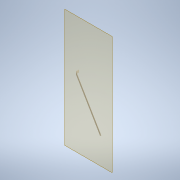
# Autodesk Inventor part: cover_inside_support_1
Saved by Autodesk Inventor 2021 (Build 250183000, 183)
## iProperties
Created: 2021-06-25
Part Number: cover_inside_support_1
Material: Generic
Document SubType Name: Modeling
Density: 1 g/cm^3
Appearance: Default
Autodesk Inventor part; units mm, degrees
ref_plane "YZ Plane" through (0, 0, 0) normal (1, 0, 0) x (0, 1, 0)
ref_plane "XZ Plane" through (0, 0, 0) normal (0, 1, 0) x (-1, 0, 0)
ref_plane "XY Plane" through (0, 0, 0) normal (0, 0, 1) x (1, 0, 0)
ref_plane "Work Plane1" through (0, 0, 0) normal (0, 0, 1) x (1, 0, 0)
sketch "Sketch1" plane through (0, 0, 0) normal (0, 0, 1) x (1, 0, 0)
  line L0 (180, 1409.2846) -> (716.3958, 495.0201)
  line L1 (180, 1350) -> (690.5204, 479.8391)
  line L2 (716.3958, 495.0201) -> (690.5204, 479.8391)
  line L3 (180, 1409.2846) -> (180, 1350)
  point P0 (0, 0)
  dimension "d0" = 30
  dimension "d2" = 180
  dimension "d3" = 1350
  dimension "d4" = 149.6
  dimension "d5" = 1060
  constraints: 8 end point, 2 perpendicular, 1 vertical
  measures "d0" distance of L0.end L1.end
  measures "d2" distance from line of point (0, 0) L3
  measures "d3" vertical distance of point (0, 0) L1.start
  measures "d4" angle of L1 L3
  measures "d5" distance of L0.start L0.end
extrude "Extrusion1" add sketch "Sketch1" against normal blind 6
sketch "Sketch2" plane through (0, 0, 0) normal (0, 0, 1) x (1, 0, 0)
  line L0 (843.3143, 1707.8077) -> (86.6419, 1707.8077)
  line L1 (86.6419, 1707.8077) -> (86.6419, 311.9107)
  line L2 (86.6419, 311.9107) -> (843.3143, 311.9107)
  line L3 (843.3143, 311.9107) -> (843.3143, 1707.8077)
  point P0 (0, 0)
  constraints: 8 end point, 2 parallel, 1 horizontal, 1 perpendicular
extrude "Extrusion2" cut sketch "Sketch2" against normal blind 3
sketch "Sketch3" plane through (0, 0, -6) normal (0, 0, -1) x (-1, 0, 0)
  line L0 (-690.5204, 479.8391) -> (-180, 1350) projected
  line L1 (-183.1729, 1344.5919) -> (-186.1729, 1344.5919)
  line L2 (-186.1729, 1344.5919) -> (-186.1729, 1403.4543)
  line L3 (-186.1729, 1403.4543) -> (-183.1729, 1403.4543)
  line L4 (-183.1729, 1403.4543) -> (-183.1729, 1344.5919)
  point P0 (0, 0)
  dimension "d10" = 3
  constraints: 8 end point, 2 parallel, 1 horizontal, 1 perpendicular, 1 point on line
  measures "d10" distance between parallel lines of L2 L4
extrude "Extrusion3" add sketch "Sketch3" along normal blind 60
fillet "Fillet1" radius 6 2 edges at (716.3958, 495.0201, -4.5) (690.5204, 479.8391, -4.5)
sketch "Sketch4" plane through (0, 0, -6) normal (0, 0, -1) x (-1, 0, 0)
  line L0 (-183.1729, 1403.4543) -> (-183.1729, 1344.5919) projected
  line L1 (-183.1729, 1403.4543) -> (-183.1729, 1344.5919)
  line L2 (-183.1729, 1403.4543) -> (-186.6492, 1397.5292)
  line L3 (-180, 1409.2846) -> (-183.4206, 1403.4543) projected
  line L4 (-186.6492, 1397.5292) -> (-186.6492, 1414.0356)
  line L5 (-186.6492, 1414.0356) -> (-167.7898, 1414.0356)
  line L6 (-167.7898, 1414.0356) -> (-167.7898, 1340.5391)
  line L7 (-167.7898, 1340.5391) -> (-183.1729, 1340.5391)
  line L8 (-183.1729, 1340.5391) -> (-183.1729, 1344.5919)
  point P0 (0, 0)
  constraints: 14 end point, 4 perpendicular, 1 parallel, 1 vertical
extrude "Extrusion4" cut sketch "Sketch4" along normal blind 90 and the other way blind 45
fillet "Fillet2" radius 2 2 edges at (183.1729, 1403.4543, -34.5) (186.1729, 1371.4664, -6)
sketch "Sketch5" plane through (183.1729, 1344.5919, -66) normal (-1, 0, 0) x (0, 0, 1)
  circle A0 centre (11.2, 32.2) radius 5
  line L0 (63, 52.017) -> (63, 0) projected
  line L1 (60, 0) -> (0, 0) projected
  point P0 (66, -1344.5919)
  dimension "d19" = 51.8
  dimension "d20" = 32.2
  dimension "d21" = 10
  constraints: 1 centre point
  measures "d19" distance from line of L0 A0.centre
  measures "d20" distance from line of L1 A0.centre
  measures "d21" diameter of A0
extrude "Extrusion5" cut sketch "Sketch5" against normal blind 10
sketch "Sketch6" plane through (0, 0, -3) normal (0, 0, 1) x (1, 0, 0)
  circle A0 centre (689.5422, 511.1487) radius 5
  line L0 (186.6492, 1397.9514) -> (713.3596, 500.1952) projected
  line L1 (711.2207, 491.9839) -> (695.6955, 482.8753) projected
  point P0 (0, 0)
  dimension "d24" = 10
  dimension "d25" = 15
  dimension "d26" = 27.5
  constraints: 1 centre point
  measures "d24" diameter of A0
  measures "d25" distance from line of A0.centre L0
  measures "d26" distance from line of L1 A0.centre
extrude "Extrusion6" cut sketch "Sketch6" against normal blind 10
body "Solid1"
